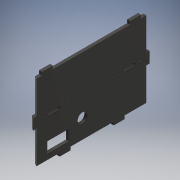
# Autodesk Inventor part: BA16
Saved by Autodesk Inventor 2017 (Build 210142000, 142)
## iProperties
Created: 2019-05-31
Part Number: BA16
Material: Polyethylene, High Density
Document SubType Name: Modeling
Designer: Dell
Density: 0.952 g/cm^3
Appearance: Smooth - Black
Mass: 274.487 g
Surface Area: 980.451 cm^2
Volume: 288.326 cm^3
Author: Dell
Autodesk Inventor part; units mm, degrees
ref_plane "YZ Plane" through (0, 0, 0) normal (1, 0, 0) x (0, 1, 0)
ref_plane "XZ Plane" through (0, 0, 0) normal (0, 1, 0) x (-1, 0, 0)
ref_plane "XY Plane" through (0, 0, 0) normal (0, 0, 1) x (1, 0, 0)
sketch "Sketch1" plane through (0, 0, 0) normal (0, 0, 1) x (1, 0, 0)
  line L0 (0, 0) -> (0, -195.6092) construction
  line L1 (0, -195.6092) -> (262.89, -347.3888) construction
  line L2 (262.89, -347.3888) -> (525.78, -195.6092) construction
  line L3 (525.78, -195.6092) -> (525.78, 0) construction
  line L4 (525.78, 0) -> (0, 0) construction
  line L5 (101.6, -254.268) -> (101.6, 0)
  line L6 (101.6, 0) -> (107.95, 0)
  line L7 (107.95, -257.9342) -> (101.6, -254.268)
  line L8 (107.95, 0) -> (107.95, -257.9342)
  point P0 (262.89, 0)
  dimension "d0" = 525.78
  dimension "d1" = 195.6092
  dimension "d2" = 120
  dimension "d3" = 6.35
  dimension "d4" = 101.6
  constraints: 18 end point, 4 point on line, 3 perpendicular, 1 collinear, 1 horizontal alignment, 1 midpoint, 1 parallel, 1 vertical, 1 vertical alignment
  measures "d0" distance of L3.end L0.start
  measures "d1" distance of L0.start L0.end
  measures "d2" angle of L2 L1
  measures "d3" distance between parallel lines of L5 L8
  measures "d4" distance between parallel lines of L0 L5
extrude "Extrusion1" add sketch "Sketch1" along normal blind 177.8
sketch "Sketch2" plane through (107.95, -257.9342, 0) normal (1, 0, 0) x (0, 0, -1)
  line L0 (0, 257.9342) -> (-177.8, 257.9342) projected
  line L1 (-101.6, 257.9342) -> (-76.2, 257.9342)
  line L2 (-76.2, 257.9342) -> (-76.2, 265.5542)
  line L3 (-76.2, 265.5542) -> (-101.6, 265.5542)
  line L4 (-101.6, 265.5542) -> (-101.6, 257.9342)
  line L5 (0, 3.6662) -> (-177.8, 3.6662) projected
  line L6 (-101.6, 3.6662) -> (-76.2, 3.6662)
  line L7 (-76.2, 3.6662) -> (-76.2, -7.62)
  line L8 (-76.2, -7.62) -> (-101.6, -7.62)
  line L9 (-101.6, -7.62) -> (-101.6, 3.6662)
  line L10 (0, 0) -> (-177.8, 0) projected
  point P0 (-88.9, 257.9342)
  point P1 (-88.9, 3.6662)
  dimension "d7" = 25.4
  dimension "d8" = 7.62
  dimension "d9" = 7.62
  constraints: 16 end point, 4 midpoint, 4 parallel, 2 horizontal, 2 perpendicular, 2 point on line, 1 vertical alignment
  measures "d7" distance of L3.end L2.end
  measures "d8" distance of L2.end L1.end
  measures "d9" distance between parallel lines of L8 L10
extrude "Extrusion2" add sketch "Sketch2" against normal blind 6.35
sketch "Sketch3" plane through (0, 0, 177.8) normal (0, 0, 1) x (1, 0, 0)
  line L0 (101.6, -254.268) -> (107.95, -257.9342) projected
  line L1 (107.95, -265.5542) -> (101.6, -265.5542) projected
  line L2 (107.95, -265.5542) -> (101.6, -261.888)
  line L3 (101.6, -265.5542) -> (101.6, -254.268) projected
  line L4 (101.6, -261.888) -> (101.6, -265.5542)
  point P0 (0, 0)
  constraints: 4 end point, 1 collinear, 1 parallel
extrude "Extrusion3" cut sketch "Sketch3" along normal through all both and the other way through all
sketch "Sketch4" plane through (101.6, -254.268, 0) normal (-1, 0, 0) x (0, 0, 1)
  line L0 (0, 203.468) -> (-7.62, 203.468)
  line L1 (-7.62, 203.468) -> (-7.62, 178.068)
  line L2 (-7.62, 178.068) -> (0, 178.068)
  line L3 (0, 178.068) -> (0, 203.468)
  line L4 (0, 0) -> (0, 254.268) projected
  line L5 (0, 76.468) -> (-7.62, 76.468)
  line L6 (-7.62, 76.468) -> (-7.62, 51.068)
  line L7 (-7.62, 51.068) -> (0, 51.068)
  line L8 (0, 51.068) -> (0, 76.468)
  line L9 (0, 254.268) -> (76.2, 254.268) projected
  dimension "d14" = 7.62
  dimension "d15" = 25.4
  dimension "d16" = 25.4
  dimension "d17" = 50.8
  dimension "d18" = 101.6
  constraints: 16 end point, 4 parallel, 2 horizontal, 2 perpendicular, 2 point on line, 1 vertical alignment
  measures "d14" distance of L0.start L0.end
  measures "d15" distance of L0.end L1.end
  measures "d16" distance of L5.end L6.end
  measures "d17" distance from line of L9 L0.end
  measures "d18" distance of L1.end L5.end
extrude "Extrusion4" add sketch "Sketch4" against normal blind 6.35
sketch "Sketch5" plane through (107.95, -257.9342, 177.8) normal (1, 0, 0) x (0, 0, -1)
  line L0 (165.1, 25.4) -> (139.7, 25.4)
  line L1 (139.7, 25.4) -> (139.7, 76.2)
  line L2 (139.7, 76.2) -> (165.1, 76.2)
  line L3 (165.1, 76.2) -> (165.1, 25.4)
  line L4 (177.8, 54.7342) -> (177.8, 0) projected
  line L5 (177.8, 0) -> (101.6, 0) projected
  point P0 (177.8, 257.9342)
  dimension "d21" = 25.4
  dimension "d22" = 50.8
  dimension "d23" = 12.7
  dimension "d24" = 25.4
  constraints: 8 end point, 2 parallel, 1 horizontal, 1 perpendicular
  measures "d21" distance of L1.end L2.end
  measures "d22" distance of L0.end L1.end
  measures "d23" distance between parallel lines of L4 L3
  measures "d24" distance between parallel lines of L5 L0
extrude "Extrusion5" cut sketch "Sketch5" against normal through all
sketch "Sketch6" plane through (101.6, -254.268, 177.8) normal (-1, 0, 0) x (0, 0, 1)
  line L0 (0, 254.268) -> (0, 0) projected
  line L1 (0, 241.568) -> (7.62, 241.568)
  line L2 (7.62, 241.568) -> (7.62, 216.168)
  line L3 (7.62, 216.168) -> (0, 216.168)
  line L4 (0, 216.168) -> (0, 241.568)
  line L5 (0, 34.4338) -> (7.62, 34.4338)
  line L6 (7.62, 34.4338) -> (7.62, 9.0338)
  line L7 (7.62, 9.0338) -> (0, 9.0338)
  line L8 (0, 9.0338) -> (0, 34.4338)
  line L9 (-76.2, 254.268) -> (0, 254.268) projected
  line L10 (-76.2, 0) -> (0, 0) projected
  point P0 (-177.8, 254.268)
  dimension "d27" = 7.62
  dimension "d28" = 25.4
  dimension "d29" = 25.4
  dimension "d30" = 12.7
  dimension "d34" = 181.7342
  constraints: 16 end point, 4 parallel, 2 horizontal, 2 perpendicular, 2 point on line, 1 vertical alignment
  measures "d27" distance of L2.end L3.end
  measures "d28" distance of L1.end L2.end
  measures "d29" distance of L5.end L6.end
  measures "d30" distance between parallel lines of L9 L1
  measures "d34" distance between parallel lines of L5 L3
extrude "Extrusion6" add sketch "Sketch6" against normal blind 6.35
sketch "Sketch7" plane through (101.6, -254.268, 101.6) normal (-1, 0, 0) x (0, 0, 1)
  line L0 (-6.35, 228.868) -> (-12.7, 228.868)
  line L1 (-12.7, 228.868) -> (-12.7, 203.468)
  line L2 (-12.7, 203.468) -> (-6.35, 203.468)
  line L3 (-6.35, 203.468) -> (-6.35, 228.868)
  line L4 (-6.35, 51.068) -> (-12.7, 51.068)
  line L5 (-12.7, 51.068) -> (-12.7, 25.668)
  line L6 (-12.7, 25.668) -> (-6.35, 25.668)
  line L7 (-6.35, 25.668) -> (-6.35, 51.068)
  line L8 (-6.35, 216.168) -> (-6.35, 38.368) construction
  line L9 (76.2, 216.168) -> (76.2, 34.4338) projected
  line L10 (-101.6, 203.468) -> (-101.6, 254.268) projected
  line L11 (0, 254.268) -> (76.2, 254.268) projected
  point P0 (-6.35, 127.268)
  point P1 (76.2, 125.3009)
  dimension "d35" = 6.35
  dimension "d36" = 25.4
  dimension "d37" = 6.35
  dimension "d38" = 25.4
  dimension "d39" = 177.8
  dimension "d40" = 88.9
  dimension "d43" = 25.4
  constraints: 18 end point, 4 midpoint, 4 parallel, 2 horizontal, 2 perpendicular, 1 point on line
  measures "d35" distance of L2.end L1.end
  measures "d36" distance of L1.end L0.end
  measures "d37" distance of L6.end L5.end
  measures "d38" distance of L5.end L4.end
  measures "d39" distance of L8.start L8.end
  measures "d40" distance between parallel lines of L10 L1
  measures "d43" distance from line of L11 L0.start
extrude "Extrusion7" cut sketch "Sketch7" against normal through all
sketch "Sketch8" plane through (101.6, -254.268, 101.6) normal (-1, 0, 0) x (0, 0, 1)
  circle A0 centre (-9.525, 176.1009) radius 2.25
  circle A1 centre (-9.525, 74.5009) radius 2.25
  line L0 (-9.525, 176.1009) -> (-9.525, 74.5009) construction
  line L1 (-6.35, 203.468) -> (-12.7, 203.468) projected
  line L2 (76.2, 216.168) -> (76.2, 34.4338) projected
  circle A2 centre (-9.525, 241.568) radius 2.25
  circle A3 centre (-9.525, 12.834) radius 2.25
  line L3 (-12.7, 228.868) -> (-6.35, 228.868) projected
  line L4 (-9.525, 228.868) -> (-9.525, 254.268) construction
  line L5 (-12.7, 25.668) -> (-6.35, 25.668) projected
  line L6 (-9.525, 25.668) -> (-9.525, 0) construction
  point P0 (-101.6, 254.268)
  point P1 (-9.525, 203.468)
  point P2 (-9.525, 125.3009)
  point P3 (76.2, 125.3009)
  point P4 (0, 254.268)
  point P5 (0, 0)
  dimension "d44" = 4.5
  dimension "d45" = 4.5
  dimension "d46" = 101.6
  dimension "d47" = 4.5
  dimension "d48" = 4.5
  constraints: 7 midpoint, 6 end point, 4 centre point, 3 horizontal alignment, 3 vertical, 2 coincident, 1 vertical alignment
  measures "d44" diameter of A0
  measures "d45" diameter of A1
  measures "d46" distance of L0.start L0.end
  measures "d47" diameter of A2
  measures "d48" diameter of A3
extrude "Extrusion8" cut sketch "Sketch8" against normal through all
sketch "Sketch9" plane through (107.95, 7.62, 101.6) normal (1, 0, 0) x (0, 0, -1)
  circle A0 centre (57.15, -157.5822) radius 11.5
  line L0 (101.6, -7.62) -> (25.4, -7.62) projected
  line L1 (101.6, -83.82) -> (101.6, -185.42) projected
  dimension "d51" = 23
  dimension "d52" = 149.9622
  dimension "d53" = 44.45
  constraints: 1 centre point
  measures "d51" diameter of A0
  measures "d52" distance from line of L0 A0.centre
  measures "d53" distance from line of L1 A0.centre
extrude "Extrusion9" cut sketch "Sketch9" against normal through all
equation "\"d3\" = Panel_Thickness"
equation "\"d8\" = Panel_Thickness + Fit_Tolerance"
equation "\"d9\" = Panel_Thickness + Fit_Tolerance"
equation "\"d10\" = Panel_Thickness"
equation "\"d14\" = Panel_Thickness + Fit_Tolerance"
equation "\"d19\" = Panel_Thickness"
equation "\"d25\" = Panel_Thickness"
equation "\"d27\" = Panel_Thickness + Fit_Tolerance"
equation "\"d32\" = Panel_Thickness"
equation "\"d35\" = Panel_Thickness"
equation "\"d37\" = Panel_Thickness"
equation "\"d41\" = Panel_Thickness"
equation "\"d49\" = Panel_Thickness"
equation "\"d54\" = Panel_Thickness"
equation "\"Panel_Thickness\" = 6.35"
equation "\"Fit_Tolerance\" = 1.27"
equation "\"Tool_Dia\" = 6.35"
body "Solid1"
